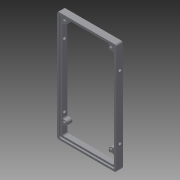
# Autodesk Inventor part: RahmenV05_BOT
Saved by Autodesk Inventor 2015 (Build 190159000, 159)
## iProperties
Created: 2016-07-21
Part Number: RahmenV05_BOT
Material: Generic
Document SubType Name: Modeling
Designer: spichelh
Density: 1 g/cm^3
Appearance: Default
Author: spichelh
Autodesk Inventor part; units mm, degrees
ref_plane "YZ Plane" through (0, 0, 0) normal (1, 0, 0) x (0, 1, 0)
ref_plane "XZ Plane" through (0, 0, 0) normal (0, 1, 0) x (-1, 0, 0)
ref_plane "XY Plane" through (0, 0, 0) normal (0, 0, 1) x (1, 0, 0)
sketch "Sketch1" plane through (0, 0, 0) normal (0, 1, 0) x (-1, 0, 0)
  line L0 (29.575, 58.88) -> (-29.575, 58.88)
  line L1 (-31.575, 56.88) -> (-31.575, -56.88)
  line L2 (-29.575, -58.88) -> (29.575, -58.88)
  line L3 (31.575, -56.88) -> (31.575, 56.88)
  line L4 (21.765, 52.07) -> (27.765, 52.07) construction
  line L5 (0, 0) -> (-80.4548, 0) construction
  line L6 (0, 0) -> (0, 46.6746) construction
  line L7 (28.575, 55.88) -> (-28.575, 55.88) construction
  line L8 (-28.575, 55.88) -> (-28.575, -55.88) construction
  line L9 (-28.575, -55.88) -> (28.575, -55.88) construction
  line L10 (28.575, -55.88) -> (28.575, 55.88) construction
  circle A0 centre (24.765, 52.07) radius 1.5 construction
  circle A1 centre (-24.765, 52.07) radius 1.5 construction
  circle A2 centre (24.765, -41.91) radius 3.8303 construction
  circle A3 centre (-24.765, -41.91) radius 3.8303 construction
  line L11 (20.265, 54.88) -> (-20.265, 54.88)
  line L12 (-25.575, -54.88) -> (25.575, -54.88)
  line L13 (28.575, 55.88) -> (-28.575, -55.88) construction
  line L14 (28.575, -55.88) -> (-28.575, 55.88) construction
  arc A4 (25.575, -54.88) -> (27.575, -52.88) centre (25.575, -52.88) ccw
  arc A5 (-27.575, -52.88) -> (-25.575, -54.88) centre (-25.575, -52.88) ccw
  arc A6 (-29.575, 58.88) -> (-31.575, 56.88) centre (-29.575, 56.88) ccw
  arc A7 (31.575, 56.88) -> (29.575, 58.88) centre (29.575, 56.88) ccw
  arc A8 (29.575, -58.88) -> (31.575, -56.88) centre (29.575, -56.88) ccw
  arc A9 (-31.575, -56.88) -> (-29.575, -58.88) centre (-29.575, -56.88) ccw
  circle A10 centre (24.765, 52.07) radius 1.5
  line L15 (24.765, 49.57) -> (25.575, 49.57)
  line L16 (22.265, 52.07) -> (22.265, 52.88)
  arc A11 (27.575, 47.57) -> (25.575, 49.57) centre (25.575, 47.57) ccw
  arc A12 (22.265, 52.88) -> (20.265, 54.88) centre (20.265, 52.88) ccw
  circle A13 centre (-24.765, 52.07) radius 1.5 construction
  circle A14 centre (-24.765, 52.07) radius 1.5
  arc A15 (-24.765, 49.57) -> (-22.265, 52.07) centre (-24.765, 52.07) ccw
  arc A16 (-25.575, 49.57) -> (-27.575, 47.57) centre (-25.575, 47.57) ccw
  arc A17 (-20.265, 54.88) -> (-22.265, 52.88) centre (-20.265, 52.88) ccw
  line L17 (-24.765, 49.57) -> (-25.575, 49.57)
  line L18 (-22.265, 52.07) -> (-22.265, 52.88)
  arc A18 (22.265, 52.07) -> (24.765, 49.57) centre (24.765, 52.07) ccw
  circle A19 centre (24.765, -41.91) radius 1.5
  circle A20 centre (-24.765, -41.91) radius 1.5
  arc A21 (-24.765, -44.41) -> (-24.765, -39.41) centre (-24.765, -41.91) ccw
  line L19 (-24.765, -44.41) -> (-25.575, -44.41)
  line L20 (-24.765, -39.41) -> (-25.575, -39.41)
  line L21 (-27.575, 47.57) -> (-27.575, -37.41)
  line L22 (-27.575, -46.41) -> (-27.575, -52.88)
  arc A22 (-27.575, -37.41) -> (-25.575, -39.41) centre (-25.575, -37.41) ccw
  arc A23 (-25.575, -44.41) -> (-27.575, -46.41) centre (-25.575, -46.41) ccw
  line L23 (24.765, -44.41) -> (25.575, -44.41)
  line L24 (24.765, -39.41) -> (25.575, -39.41)
  arc A24 (25.575, -39.41) -> (27.575, -37.41) centre (25.575, -37.41) ccw
  arc A25 (27.575, -46.41) -> (25.575, -44.41) centre (25.575, -46.41) ccw
  line L25 (27.575, -52.88) -> (27.575, -46.41)
  line L26 (27.575, -37.41) -> (27.575, 47.57)
  arc A26 (24.765, -39.41) -> (24.765, -44.41) centre (24.765, -41.91) ccw
  point P0 (31.575, 58.88)
  point P1 (-31.575, -58.88)
  point P2 (-31.575, 58.88)
  point P3 (31.575, -58.88)
  point P4 (-27.575, 54.88)
  dimension "d77" = 57.15
  dimension "d78" = 3.81
  dimension "d79" = 3.81
  dimension "d80" = 3.81
  dimension "d81" = 3.81
  dimension "d82" = 3
  dimension "d85" = 111.76
  dimension "d88" = 3.81
  dimension "d100" = 1
  dimension "d101" = 3
  dimension "d104" = 1
  dimension "d107" = 3
  dimension "d109" = 3
  dimension "d122" = 3
  dimension "d123" = 2
  dimension "d132" = 2
  dimension "d145" = 2
  dimension "d150" = 2.5
  dimension "d151" = 3
  dimension "d152" = 3
  dimension "d154" = 5
  dimension "d155" = 2
  dimension "d156" = 1
  dimension "d157" = 12.97
  constraints: 54 end point, 36 point on circle, 29 tangent, 27 centre point, 20 symmetric about line, 10 point on line, 9 parallel, 9 perpendicular, 8 coincident, 7 equal radius, 6 horizontal, 2 midpoint, 1 vertical, 7 other
  measures "d77" distance of L7.start L7.end
  measures "d78" distance from line of L8 A1.centre
  measures "d79" distance from line of L7 A1.centre
  measures "d80" distance from line of L7 A0.centre
  measures "d81" distance from line of L10 A0.centre
  measures "d82" diameter of A0
  measures "d85" distance of L9.end L7.start
  measures "d88" distance from line of L10 A2.centre
  measures "d100" distance between parallel lines of L7 L11
  measures "d101" distance between parallel lines of L0 L7
  measures "d104" distance between parallel lines of L9 L12
  measures "d107" distance between parallel lines of L2 L9
  measures "d109" distance between parallel lines of L3 L10
  measures "d122" distance between parallel lines of L8 L1
  measures "d123" radius of A4
  measures "d132" radius of A6
  measures "d145" radius of A11
  measures "d150" radius of A18
  measures "d151" diameter of A19
  measures "d152" diameter of A20
  measures "d154" diameter of A21
  measures "d155" radius of A22
  measures "d156" distance between parallel lines of L8 L21
  measures "d157" distance from line of L12 A3.centre
extrude "Extrusion1" add sketch "Sketch1" along normal blind 7
sketch "Sketch2" plane through (0, 0, 0) normal (0, -1, 0) x (1, 0, 0)
  line L0 (-27.575, 56.88) -> (27.575, 56.88)
  line L1 (29.575, 54.88) -> (29.575, -54.88)
  line L2 (27.575, -56.88) -> (-27.575, -56.88)
  line L3 (-29.575, -54.88) -> (-29.575, 54.88)
  line L4 (29.575, 56.88) -> (-29.575, -56.88) construction
  line L5 (29.575, -56.88) -> (-29.575, 56.88) construction
  arc A0 (29.575, 54.88) -> (27.575, 56.88) centre (27.575, 54.88) ccw
  arc A1 (-27.575, 56.88) -> (-29.575, 54.88) centre (-27.575, 54.88) ccw
  arc A2 (-29.575, -54.88) -> (-27.575, -56.88) centre (-27.575, -54.88) ccw
  arc A3 (27.575, -56.88) -> (29.575, -54.88) centre (27.575, -54.88) ccw
  circle A4 centre (-24.765, 52.07) radius 1.5 projected
  point P0 (0, 0)
  dimension "d26" = 59.15
  dimension "d27" = 113.76
  dimension "d131" = 2
  constraints: 12 end point, 8 point on circle, 8 point on line, 8 tangent, 4 centre point, 3 equal radius, 2 midpoint, 2 parallel, 1 horizontal, 1 perpendicular
  measures "d26" distance of L5.end L4.start
  measures "d27" distance of L4.start L5.start
  measures "d131" radius of A0
extrude "Extrusion2" cut sketch "Sketch2" against normal blind 1.6
sketch "Sketch5" plane through (-31.575, 0, -56.88) normal (-1, 0, 0) x (0, 0, 1)
  circle A0 centre (23, 4) radius 1.5
  circle A1 centre (90.76, 4) radius 1.5
  line L0 (10.47, 7) -> (4, 7) projected
  line L1 (115.76, 0) -> (115.76, 7) projected
  line L2 (-2, 0) -> (-2, 7) projected
  circle A2 centre (90.76, 5.5) radius 1.5
  line L3 (92.26, 4) -> (92.26, 5.5)
  line L4 (90.76, 4) -> (90.76, 5.5) construction
  line L5 (89.26, 5.5) -> (89.26, 4)
  point P0 (56.88, 0)
  point P1 (109.76, 7)
  point P2 (104.45, 7)
  dimension "d133" = 3
  dimension "d134" = 3
  dimension "d135" = 3
  dimension "d136" = 3
  dimension "d137" = 25
  dimension "d138" = 25
  dimension "d141" = 3
  dimension "d142" = 1.5
  constraints: 6 end point, 5 point on circle, 3 centre point, 3 vertical, 2 tangent
  measures "d133" diameter of A0
  measures "d134" diameter of A1
  measures "d135" distance from line of L0 A0.centre
  measures "d136" distance from line of L0 L4.start
  measures "d137" distance from line of L4.start L1
  measures "d138" distance from line of L2 A0.centre
  measures "d141" diameter of A2
  measures "d142" distance of L4.start L4.end
extrude "Extrusion5" cut sketch "Sketch5" against normal blind 70 contours A0 | A1 A2 | A1 A2 picked at (90.702, 3.0107) picked at (90.702, 4.5034)
sketch "Sketch6" plane through (0, 1.6, 0) normal (0, -1, 0) x (1, 0, 0)
  circle A0 centre (-24.765, 52.07) radius 1.5 projected
  circle A1 centre (24.765, 52.07) radius 1.5 projected
  circle A2 centre (24.765, -41.91) radius 1.5 projected
  circle A3 centre (-24.765, -41.91) radius 1.5 projected
  point P0 (0, 0)
extrude "Extrusion6" add sketch "Sketch6" along normal blind 1.6 and the other way blind 5.4
body "Solid1"
